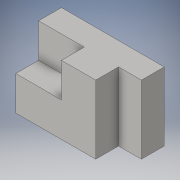
# Autodesk Inventor part: Figure 7_27_3
Saved by Autodesk Inventor 2016 (Build 200138000, 138)
## iProperties
Created: 2016-07-18
Part Number: Figure 7_27_3
Material: Generic
Document SubType Name: Modeling
Designer: cfkguest
Density: 1 g/cm^3
Appearance: Default
Author: cfkguest
Autodesk Inventor part; units mm, degrees
ref_plane "YZ Plane" through (0, 0, 0) normal (1, 0, 0) x (0, 1, 0)
ref_plane "XZ Plane" through (0, 0, 0) normal (0, 1, 0) x (-1, 0, 0)
ref_plane "XY Plane" through (0, 0, 0) normal (0, 0, 1) x (1, 0, 0)
sketch "Sketch1" plane through (0, 0, 0) normal (0, 0, 1) x (1, 0, 0)
  line L0 (-25.4, 15.1328) -> (31.75, 15.1328)
  line L1 (31.75, 15.1328) -> (31.75, -22.9672)
  line L2 (31.75, -22.9672) -> (-25.4, -22.9672)
  line L3 (-25.4, -22.9672) -> (-25.4, 15.1328)
  point P0 (0, 0)
  dimension "d0" = 57.15
  dimension "d1" = 38.1
  constraints: 8 end point, 2 parallel, 1 horizontal, 1 perpendicular
  measures "d0" distance of L1.end L2.end
  measures "d1" distance of L2.end L0.start
extrude "Extrusion1" add sketch "Sketch1" along normal blind 25.4
sketch "Sketch2" plane through (0, 0, 25.4) normal (0, 0, 1) x (1, 0, 0)
  line L0 (-25.4, 15.1328) -> (-25.4, -22.9672) projected
  line L1 (31.75, 15.1328) -> (-25.4, 15.1328) projected
  line L2 (-25.4, -3.9172) -> (0, -3.9172)
  line L3 (0, -3.9172) -> (0, 15.1328)
  line L4 (0, 15.1328) -> (-25.4, 15.1328)
  line L5 (-25.4, 15.1328) -> (-25.4, -3.9172)
  point P0 (0, 0)
  dimension "d4" = 19.05
  dimension "d5" = 25.4
  constraints: 8 end point, 2 parallel, 1 horizontal, 1 midpoint, 1 perpendicular, 1 point on line
  measures "d4" distance of L2.end L3.end
  measures "d5" distance of L2.start L2.end
extrude "Extrusion2" cut sketch "Sketch2" against normal blind 12.7
sketch "Sketch3" plane through (31.75, -22.9672, 0) normal (1, 0, 0) x (0, 0, -1)
  line L0 (0, 0) -> (-25.4, 0) projected
  line L1 (0, 38.1) -> (-25.4, 38.1) projected
  line L2 (-12.7, 0) -> (-25.4, 0)
  line L3 (-25.4, 0) -> (-25.4, 38.1)
  line L4 (-25.4, 38.1) -> (-12.7, 38.1)
  line L5 (-12.7, 38.1) -> (-12.7, 0)
  point P0 (0, 22.9672)
  dimension "d8" = 12.7
  constraints: 8 end point, 2 parallel, 1 horizontal, 1 midpoint, 1 perpendicular
  measures "d8" distance between parallel lines of L3 L5
extrude "Extrusion3" cut sketch "Sketch3" against normal blind 12.7
body "Solid1"
